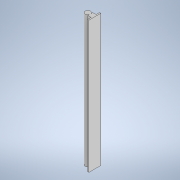
# Autodesk Inventor part: Riel
Saved by Autodesk Inventor 2021 (Build 250183000, 183)
## iProperties
Created: 2022-02-08
Part Number: Riel
Material: Generic
Document SubType Name: Modeling
Designer: deuts
Density: 1 g/cm^3
Appearance: Default
Author: deuts
Autodesk Inventor part; units mm, degrees
ref_plane "YZ Plane" through (0, 0, 0) normal (1, 0, 0) x (0, 1, 0)
ref_plane "XZ Plane" through (0, 0, 0) normal (0, 1, 0) x (-1, 0, 0)
ref_plane "XY Plane" through (0, 0, 0) normal (0, 0, 1) x (1, 0, 0)
sketch "Sketch1" plane through (0, 0, 0) normal (0, 1, 0) x (-1, 0, 0)
  line L0 (-2.5, 22.5) -> (2.5, 22.5)
  line L1 (2.5, -22.5) -> (-2.5, -22.5)
  line L2 (-2.5, -22.5) -> (-2.5, 22.5)
  line L3 (15.2, -9.5) -> (2.5, -9.5)
  line L4 (-2.5, -9.5) -> (-2.5, 9.5)
  line L5 (2.5, 9.5) -> (15.2, 9.5)
  arc A0 (15.2, -3.6756) -> (15.2, 3.6756) centre (24.5, 0) ccw
  line L6 (15.2, 9.5) -> (15.2, 3.6756)
  line L7 (15.2, -3.6756) -> (15.2, -9.5)
  line L8 (2.5, 22.5) -> (2.5, 9.5)
  line L9 (2.5, -9.5) -> (2.5, -22.5)
  point P0 (0, 0)
  point P1 (2.5, 0)
  constraints: 20 end point, 6 parallel, 3 perpendicular, 2 horizontal, 2 point on circle, 1 centre point, 1 point on line
extrude "Extrusion1" add sketch "Sketch1" along normal blind 500
body "Solid1"
